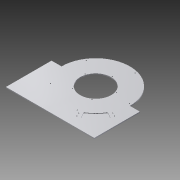
# Autodesk Inventor part: bakplate
Saved by Autodesk Inventor 2015 (Build 190159000, 159)
## iProperties
Created: 2015-02-04
Part Number: bakplate
Material: Generic
Document SubType Name: Modeling
Designer: janov_000
Density: 1 g/cm^3
Appearance: Aluminum - Flat
od: 320,000 mm
id: 150,000 mm
Author: janov_000
Autodesk Inventor part; units mm, degrees
ref_plane "YZ Plane" through (0, 0, 0) normal (1, 0, 0) x (0, 1, 0)
ref_plane "XZ Plane" through (0, 0, 0) normal (0, 1, 0) x (-1, 0, 0)
ref_plane "XY Plane" through (0, 0, 0) normal (0, 0, 1) x (1, 0, 0)
sketch "Sketch1" plane through (0, 0, 0) normal (0, 0, 1) x (1, 0, 0)
  circle A0 centre (0, 0) radius 75
  circle A1 centre (0, 0) radius 160
  arc A2 (165, 0) -> (-165, 0) centre (0, 0) ccw
  line L0 (-213, 0) -> (-213, -220)
  line L1 (-213, -220) -> (213, -220)
  line L2 (213, -220) -> (213, 0)
  line L3 (213, 0) -> (165, 0)
  line L4 (-165, 0) -> (-213, 0)
  dimension "inner_diameter" = 150
  dimension "outer_diameter" = 320
  dimension "d37" = 330
  dimension "d38" = 426
  dimension "d39" = 220
  dimension "d40" = 213
  dimension "d41" = 220
  constraints: 10 end point, 3 centre point, 3 coincident, 3 parallel, 2 horizontal, 2 perpendicular, 2 point on circle, 1 point on line
  measures "inner_diameter" diameter of A0
  measures "outer_diameter" diameter of A1
  measures "d37" diameter of A2
  measures "d38" distance of L0.end L1.end
  measures "d39" distance of L1.end L2.end
  measures "d40" distance from line of point (0, 0) L2
  measures "d41" distance of L0.start L0.end
extrude "Extrusion1" add sketch "Sketch1" along normal blind 5 contours A1 | L3 L2 L1 L0 L4 A2
sketch "Sketch2" plane through (0, 0, 5) normal (0, 0, 1) x (1, 0, 0)
  circle A0 centre (0, 0) radius 155 construction
  line L0 (0.1758, 0.0573) -> (40.2666, 149.6783) construction
  line L1 (0.1758, 0.0573) -> (-129.7335, 84.4214) construction
  line L2 (0.1758, 0.0573) -> (-120.2034, -97.4238) construction
  line L3 (0.1758, 0.0573) -> (55.6866, -144.5534) construction
  line L4 (0.1758, 0.0573) -> (154.8625, 8.1641) construction
  line L5 (0.1758, 0.0573) -> (0.1758, 154.9999) construction
  dimension "d4" = 310
  dimension "d30" = 360
  dimension "d36" = 15
  constraints: 12 end point, 8 coincident, 2 point on circle, 1 centre point, 1 vertical, 20 other
  measures "d4" diameter of A0
  measures "d36" angle of L5 L0
hole "Hole1" at (40.2666, 149.6783, 5) at (-129.7335, 84.4214, 5) at (-120.2034, -97.4238, 5) at (55.6866, -144.5534, 5) at (154.8625, 8.1641, 5) direction (0, 0, -1) diameter 4.134 depth 8 tip angle 118 thread size "M5x0.8" class "6H" standard "ANSI Metric M Profile"
sketch "Sketch3" plane through (0, 0, 5) normal (0, 0, 1) x (1, 0, 0)
  circle A0 centre (0, 0) radius 80 construction
  line L0 (0, 0) -> (0, 80) construction
  point P0 (-76.0845, 24.7214)
  point P1 (-76.0845, 24.7214)
  point P2 (-47.0228, -64.7214)
  point P3 (-47.0228, -64.7214)
  point P4 (47.0228, -64.7214)
  point P5 (47.0228, -64.7214)
  point P6 (76.0845, 24.7214)
  point P7 (76.0845, 24.7214)
  dimension "inner_holes_diameter" = 160
  dimension "d34" = 360
  constraints: 12 coincident, 2 end point, 1 vertical, 1 vertical alignment, 21 other
hole "Hole2" at (0, 80, 5) at (76.0845, 24.7214, 5) at (47.0228, -64.7214, 5) at (-47.0228, -64.7214, 5) at (-76.0845, 24.7214, 5) direction (0, 0, -1) diameter 4.134 depth 8 tip angle 118 thread size "M5x0.8" class "6H" standard "ANSI Metric M Profile"
sketch "Sketch5" plane through (0, 0, 5) normal (0, 0, 1) x (1, 0, 0)
  arc A0 (0, -160) -> (80, -138.5641) centre (0, 0) ccw construction
  line L0 (0, 0) -> (0, -160) construction
  arc A1 (104.4083, -170.584) -> (170.584, -104.4083) centre (0, 0) ccw
  line L1 (0, 0) -> (138.5641, -80) construction
  line L2 (0, 0) -> (80, -138.5641) construction
  arc A2 (138.5641, -80) -> (0, -160) centre (0, 0) ccw construction
  arc A3 (84.1622, -136.0762) -> (136.0762, -84.1622) centre (0, 0) ccw
  line L3 (82.4621, -142.8286) -> (97.4679, -168.8194)
  line L4 (142.8286, -82.4621) -> (168.8194, -97.4679)
  arc A4 (142.8286, -82.4621) -> (136.0762, -84.1622) centre (140.3286, -86.7922) ccw
  arc A5 (170.584, -104.4083) -> (168.8194, -97.4679) centre (166.3194, -101.7981) ccw
  arc A6 (97.4679, -168.8194) -> (104.4083, -170.584) centre (101.7981, -166.3194) ccw
  arc A7 (84.1622, -136.0762) -> (82.4621, -142.8286) centre (86.7922, -140.3286) ccw
  point P0 (100, -173.2051)
  point P1 (173.2051, -100)
  dimension "d50" = 320
  dimension "d51" = 200
  dimension "d52" = 30
  dimension "d53" = 30
  dimension "d54" = 5
  constraints: 20 point on circle, 10 end point, 8 centre point, 8 tangent, 4 point on line, 3 equal radius, 2 coincident, 2 collinear, 1 vertical
  measures "d50" diameter of A0
  measures "d51" radius of A1
  measures "d52" angle of L2 L1
  measures "d53" angle of L2 L0
  measures "d54" radius of A4
extrude "Extrusion3" cut sketch "Sketch5" against normal blind 3
sketch "Sketch6" plane through (0, 0, 5) normal (0, 0, 1) x (1, 0, 0)
  arc A0 (142.8286, -82.4621) -> (136.0762, -84.1622) centre (140.3286, -86.7922) ccw projected
  arc A1 (84.1622, -136.0762) -> (136.0762, -84.1622) centre (0, 0) ccw projected
  arc A2 (84.1622, -136.0762) -> (82.4621, -142.8286) centre (86.7922, -140.3286) ccw projected
  line L0 (97.4679, -168.8194) -> (82.4621, -142.8286) projected
  arc A3 (97.4679, -168.8194) -> (104.4083, -170.584) centre (101.7981, -166.3194) ccw projected
  arc A4 (104.4083, -170.584) -> (170.584, -104.4083) centre (0, 0) ccw projected
  arc A5 (170.584, -104.4083) -> (168.8194, -97.4679) centre (166.3194, -101.7981) ccw projected
  line L1 (142.8286, -82.4621) -> (168.8194, -97.4679) projected
  circle A6 centre (0, 0) radius 170 construction
  circle A7 centre (0, 0) radius 187.5 construction
  line L2 (0, 0) -> (0, -170) construction
  line L3 (0, 0) -> (79.2409, -169.9327) construction
  line L4 (0, 0) -> (169.9327, -79.2409) construction
  point P0 (71.8451, -154.0723)
  point P1 (154.0723, -71.8451)
  dimension "d57" = 340
  dimension "d58" = 375
  dimension "d59" = 25
  dimension "d60" = 40
  constraints: 6 end point, 5 point on circle, 4 coincident, 2 centre point, 2 point on line, 1 vertical
  measures "d57" diameter of A6
  measures "d58" diameter of A7
  measures "d59" angle of L3 L2
  measures "d60" angle of L4 L3
hole "Hole3" at (71.8451, -154.0723, 5) at (79.2409, -169.9327, 5) at (169.9327, -79.2409, 5) at (154.0723, -71.8451, 5) direction (0, 0, -1) diameter 4.134 end through all thread size "M5x0.8" class "6H" standard "ANSI Metric M Profile"
equation "\"inner_diameter\" = id"
equation "\"outer_diameter\" = od"
equation "\"d40\" = 0.5 * d38"
equation "\"d50\" = od"
equation "\"id\" = 150"
equation "\"od\" = 320"
body "Solid1"
